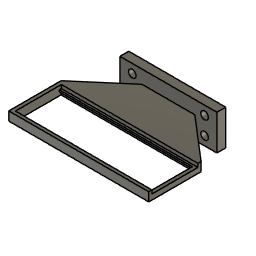
Specimen_slide_holder v2 (Autodesk Fusion 360 design; units mm, degrees)
Autodesk Fusion 360 part; units mm, degrees
note: some values were not read from the file. Set by a fixed rule: which sketch regions a step uses.
sketch "Sketch1" plane through (0, 0, 0) normal (0, 1, 0) x (1, 0, 0)
  line L0 (0, 0) -> (55, 0)
  line L1 (55, 0) -> (55, -20)
  line L2 (55, -20) -> (0, -20)
  line L3 (0, -20) -> (0, 0)
  line L4 (7, -20) -> (7, 0) construction
  line L5 (27.5, -20) -> (27.5, 0)
  line L6 (0, -10) -> (55, -10)
  line L7 (48, -20) -> (48, 0) construction
  line L8 (55, -15) -> (0, -15) construction
  circle A0 centre (7, -15) radius 2.15
  line L9 (55, -5) -> (0, -5) construction
  circle A1 centre (48, -15) radius 2.15
  circle A2 centre (7, -5) radius 2.15
  circle A3 centre (48, -5) radius 2.15
  line L10 (27.5, -10) -> (27.5, -12.5) construction
  line L11 (27.5, -12.5) -> (12.5, -12.5)
  line L12 (27.5, -12.5) -> (42.5, -12.5)
  line L13 (27.5, -7.5) -> (12.5, -7.5)
  line L14 (27.5, -7.5) -> (42.5, -7.5)
  line L15 (42.5, -12.5) -> (42.5, -7.5)
  line L16 (12.5, -12.5) -> (12.5, -7.5)
  dimension "d1" = 55
  dimension "d2" = 20
  dimension "d3" = 7
  dimension "d4" = 5
  dimension "d6" = 4.3
  dimension "d7" = 2.5
  dimension "d8" = 15
  dimension "d9" = 15
  constraint horizontal L0
  constraint vertical L1
  constraint horizontal L2
  constraint vertical L3
  constraint coincident L0.start L3.end
  constraint midpoint L2 L5.start
  constraint midpoint L0 L5.end
  constraint midpoint L3 L6.start
  constraint midpoint L1 L6.end
  constraint symmetric L4.start L5 L7.start
  constraint symmetric L4.end L5 L7.end
  constraint coincident L4 A0.centre
  constraint coincident L8 A0.centre
  constraint symmetric L6 L8.start L9.start
  constraint symmetric L6 L8.end L9.end
  constraint symmetric L5 A0 A1
  constraint symmetric L6 A0 A2
  constraint symmetric L6 A1 A3
  constraint midpoint L6 L10.start
  constraint perpendicular L2 L10
  constraint perpendicular L10 L11
  constraint perpendicular L10 L12
  constraint symmetric L6 L10.end L13.start
  constraint symmetric L6 L11.end L13.end
  constraint symmetric L6 L12.end L14.end
  measures "d1" distance of L0.start L0.end
  measures "d2" distance of L0.start L2.end
  measures "d6" diameter of A0
  measures "d7" distance of L10.start L10.end
  measures "d8" distance of L10.end L11.end
  measures "d9" distance of L10.end L12.end
extrude "Extrude1" add sketch "Sketch1" against normal blind 5 contours L0 L3 L5 L6 L13 L16 | L0 L1 L5 L6 L14 L15 | L2 L3 L5 L6 L11 L16 | L1 L2 L5 L6 L12 L15 makes body 1
extrude "Extrude2" add sketch "Sketch1" against normal blind 35 contours L5 L6 L14 L15 | L5 L6 L13 L16 | L5 L6 L11 L16 | L5 L6 L12 L15 bodies 1
ref_plane "WorkPlane1" through (27.5, -35, 10) normal (0, -1, 0) x (0, 0, -1)
sketch "Sketch2" plane through (0, -35, 0) normal (0, -1, 0) x (-1, 0, 0)
  line L0 (0, -20) -> (-55, -20) construction
  line L1 (-55, -20) -> (-55, 0) construction
  line L2 (-55, 0) -> (0, 0) construction
  line L3 (0, 0) -> (0, -20) construction
  line L4 (0, -10) -> (-55, -10)
  line L5 (-42.5, -12.5) -> (-42.5, -7.5) construction
  line L6 (-12.5, -7.5) -> (-12.5, -12.5) construction
  line L7 (-12.5, -12.5) -> (-42.5, -12.5) construction
  line L8 (-42.5, -7.5) -> (-12.5, -7.5) construction
  line L9 (-27.5, -20) -> (-27.5, 0) construction
  line L10 (-27.5, -10) -> (12.2, -10) construction
  line L11 (-27.5, -10) -> (-67.2, -10) construction
  line L12 (-27.5, -12.5) -> (12.2, -12.5)
  line L13 (-27.5, -12.5) -> (-67.2, -12.5)
  line L14 (-27.5, -7.5) -> (12.2, -7.5)
  line L15 (-27.5, -7.5) -> (-67.2, -7.5)
  line L16 (12.2, -12.5) -> (12.2, -7.5)
  line L17 (-67.2, -12.5) -> (-67.2, -7.5)
  line L18 (12.2, -12.5) -> (10.2, -12.5) construction
  line L19 (10.2, -12.5) -> (10.2, -7.5) construction
  line L20 (-67.2, -12.5) -> (-65.2, -12.5) construction
  line L21 (-65.2, -12.5) -> (-65.2, -7.5) construction
  point P0 (12.2, -12.5)
  dimension "d19" = 39.7
  dimension "d20" = 39.7
  dimension "d21" = 2.5
  dimension "d22" = 2
  dimension "d23" = 2
  constraint horizontal L0
  constraint vertical L1
  constraint horizontal L2
  constraint vertical L3
  constraint midpoint L3 L4.start
  constraint midpoint L1 L4.end
  constraint vertical L5
  constraint vertical L6
  constraint perpendicular L5 L7
  constraint perpendicular L6 L8
  constraint midpoint L0 L9.start
  constraint midpoint L2 L9.end
  constraint horizontal L10
  constraint midpoint L9 L10.start
  constraint perpendicular L9 L11
  constraint symmetric L4 L12.start L14.start
  constraint symmetric L4 P0 L14.end
  constraint symmetric L4 L13.end L15.end
  constraint perpendicular L16 L18
  constraint coincident L14 L19.end
  constraint perpendicular L14 L19
  constraint perpendicular L17 L20
  constraint coincident L15 L21.end
  constraint perpendicular L15 L21
  constraint coincident P0 L12.end
  measures "d19" distance of L10.start L10.end
  measures "d20" distance of L10.start L11.end
  measures "d22" distance of P0 L18.end
  measures "d23" distance of L13.end L20.end
ref_plane "WorkPlane2" through (27.5, -35, 7.5) normal (0, 0, 1) x (-1, 0, 0)
sketch "Sketch3" plane through (0, 0, 7.5) normal (0, 0, 1) x (1, 0, 0)
extrude "Extrude4" add sketch "Sketch2" along normal blind 29.7 bodies 1
sketch "Sketch4" plane through (0, 0, 12.5) normal (0, 0, 1) x (-1, 0, 0)
  line L0 (-42.5, 5) -> (-12.5, 5)
  line L1 (-12.5, 5) -> (-12.5, 35)
  line L2 (-12.5, 35) -> (12.2, 35)
  line L3 (12.2, 35) -> (12.2, 64.7)
  line L4 (12.2, 64.7) -> (-67.2, 64.7)
  line L5 (-67.2, 64.7) -> (-67.2, 35)
  line L6 (-67.2, 35) -> (-42.5, 35)
  line L7 (-42.5, 35) -> (-42.5, 5)
  line L8 (12.2, 35) -> (-67.2, 35) construction
  line L9 (-67.2, 35) -> (-67.2, 64.7) construction
  line L10 (-67.2, 64.7) -> (12.2, 64.7) construction
  line L11 (12.2, 64.7) -> (12.2, 35) construction
  line L12 (-65.2, 62.7) -> (10.2, 62.7)
  line L13 (10.2, 36) -> (-65.2, 36)
  line L14 (-27.5, 35) -> (-27.5, 64.7)
  line L15 (-65.2, 49.85) -> (10.2, 49.85)
  line L16 (10.25, 62.7) -> (10.25, 36)
  line L17 (10.25, 36) -> (10.2, 36)
  line L18 (10.25, 62.7) -> (10.2, 62.7)
  line L19 (-65.25, 62.7) -> (-65.25, 36)
  line L20 (-65.25, 62.7) -> (-65.2, 62.7)
  line L21 (-65.25, 36) -> (-65.2, 36)
  line L22 (-65.2, 61.7) -> (10.2, 61.7)
  line L23 (10.2, 61.7) -> (10.25, 61.7)
  line L24 (-65.2, 61.7) -> (-65.25, 61.7)
  line L25 (10.2, 37) -> (-65.2, 37)
  line L26 (10.2, 37) -> (10.25, 37)
  line L27 (-65.2, 37) -> (-65.25, 37)
  line L28 (10.2, 38) -> (10.25, 38)
  line L29 (-65.2, 38) -> (10.2, 38)
  line L30 (-65.2, 38) -> (-65.25, 38)
  line L31 (-65.25, 62.7) -> (-67.2, 62.7)
  line L32 (-65.25, 37) -> (-67.2, 37)
  line L33 (-42.5, 20) -> (-57.5, 35)
  line L34 (-27.5, 5) -> (-27.5, 34.5958)
  line L35 (-12.5, 20) -> (2.5, 35)
  dimension "d36" = 1
  dimension "d39" = 1
  constraint horizontal L8
  constraint vertical L9
  constraint horizontal L10
  constraint vertical L11
  constraint coincident L4.end L5.start
  constraint coincident L2.end L3.start
  constraint midpoint L8 L14.start
  constraint midpoint L10 L14.end
  constraint symmetric L13.start L14 L13.end
  constraint symmetric L12.end L14 L12.start
  constraint perpendicular L16 L17
  constraint perpendicular L16 L18
  constraint perpendicular L19 L20
  constraint perpendicular L19 L21
  constraint coincident L16 L23.end
  constraint perpendicular L16 L23
  constraint coincident L19 L24.end
  constraint perpendicular L19 L24
  constraint coincident L16 L26.end
  constraint perpendicular L16 L26
  constraint coincident L19 L27.end
  constraint perpendicular L19 L27
  constraint symmetric L15 L22.start L29.start
  constraint symmetric L15 L22.end L28.start
  constraint symmetric L15 L23.end L28.end
  constraint symmetric L15 L24.end L30.end
  constraint coincident L9 L31.end
  constraint perpendicular L9 L31
  constraint coincident L9 L32.end
  constraint perpendicular L9 L32
  constraint midpoint L7 L33.start
  constraint coincident L8 L33.end
  constraint midpoint L0 L34.start
  constraint perpendicular L8 L34
  constraint symmetric L33.start L34 L35.start
  constraint symmetric L33.end L34 L35.end
extrude "Extrude5" cut sketch "Sketch4" against normal blind 40 contours L13 L14 L19 L21 L25 L27 | L14 L19 L25 L27 L29 L30 | L12 L14 L19 L20 L22 L24 | L14 L19 L22 L24 L29 L30 | L13 L14 L16 L17 L25 L26 | L14 L16 L25 L26 L28 L29 | L12 L14 L16 L18 L22 L23 | L14 L16 L22 L23 L28 L29 bodies 1
extrude "Extrude6" add sketch "Sketch4" against normal blind 3.5 contours L13 L14 L19 L21 L25 L27 | L13 L14 L16 L17 L25 L26 bodies 1
extrude "Extrude7" add 1 faces at (40.0833, -36.6667, 9) along direction (0, 0, -1) blind 1.5 on bodies 1 bodies 1
extrude "Extrude8" add sketch "Sketch4" against normal blind 3.5 contours L14 L19 L25 L27 L29 L30 | L14 L16 L25 L26 L28 L29 bodies 1
extrude "Extrude9" cut sketch "Sketch4" against normal blind 2.5 contours L14 L19 L25 L27 L29 L30 | L14 L16 L25 L26 L28 L29 bodies 1
extrude "Extrude10" add sketch "Sketch4" against normal blind 3.5 contours L12 L14 L19 L20 L22 L24 | L12 L14 L16 L18 L22 L23 bodies 1
extrude "Extrude11" cut sketch "Sketch4" against normal blind 2.5 contours L12 L14 L19 L20 L22 L24 | L12 L14 L16 L18 L22 L23 bodies 1
sketch "Sketch5" plane through (67.2, 0, 0) normal (1, 0, 0) x (0, 1, 0)
  line L0 (-35, 7.5) -> (-35, 12.5)
  line L1 (-35, 12.5) -> (-64.7, 12.5)
  line L2 (-64.7, 12.5) -> (-64.7, 7.5)
  line L3 (-64.7, 7.5) -> (-35, 7.5)
  line L4 (-49.85, 12.5) -> (-49.85, 7.5)
  line L5 (-64.7, 10) -> (-35, 10)
  line L6 (-49.85, 10) -> (-49.85, 10.75) construction
  line L7 (-49.85, 10.75) -> (-62.7, 10.75)
  line L8 (-49.85, 9.25) -> (-62.7, 9.25)
  line L9 (-49.85, 10.75) -> (-37, 10.75)
  line L10 (-49.85, 9.25) -> (-37, 9.25)
  line L11 (-62.7, 10.75) -> (-62.7, 9.25)
  line L12 (-37, 10.75) -> (-37, 9.25)
  dimension "d51" = 0.75
  constraint midpoint L1 L4.start
  constraint midpoint L3 L4.end
  constraint midpoint L2 L5.start
  constraint midpoint L0 L5.end
  constraint midpoint L4 L6.start
  constraint perpendicular L5 L6
  constraint horizontal L7
  constraint symmetric L5 L6.end L8.start
  constraint symmetric L5 L7.end L8.end
  constraint symmetric L4 L6.end L7.start
  constraint symmetric L4 L7.end L9.end
  constraint symmetric L4 L8.start L10.start
  constraint symmetric L4 L8.end L10.end
  constraint perpendicular L8 L11
  measures "d51" distance of L6.start L6.end
extrude "Extrude12" cut sketch "Sketch5" against normal blind 2 contours L4 L5 L10 L12 | L4 L5 L9 L12 | L4 L5 L8 L11 | L4 L5 L7 L11 bodies 1
extrude "Extrude13" add 1 faces at (40.05, -62.3667, 10) along direction (0, 0, 1) blind 0.5 on bodies 1 bodies 1
extrude "Extrude14" cut 1 faces at (40.0833, -62.3667, 9) along direction (0, 0, 1) blind 0.5 on bodies 1 bodies 1
extrude "Extrude15" add 1 faces at (40.05, -37.3333, 10) along direction (0, 0, 1) blind 0.5 on bodies 1 bodies 1
extrude "Extrude16" cut 1 faces at (14.9167, -37.6667, 9) along direction (0, 0, 1) blind 0.5 on bodies 1 bodies 1
extrude "Extrude17" add 1 faces at (66.55, -45.5667, 9.25) along direction (0, 0, 1) blind 2 on bodies 1 bodies 1
extrude "Extrude18" cut sketch "Sketch4" against normal blind 2 contours L5 L19 L31 L32 bodies 1
extrude "Extrude19" add 1 faces at (65.2, -62.3667, 10.1667) along direction (1, 0, 0) blind 0.1 on bodies 1 bodies 1
extrude "Extrude20" add 1 faces at (65.2, -37.3333, 9.8333) along direction (1, 0, 0) blind 0.1 on bodies 1 bodies 1
extrude "Extrude21" cut 1 faces at (40.7167, -62.7, 11.8333) along direction (0, -1, 0) blind 0.1 on bodies 1 bodies 1
extrude "Extrude22" cut 1 faces at (40.0667, -37, 11.8333) along direction (0, 1, 0) blind 0.2 on bodies 1 bodies 1
extrude "Extrude23" cut 1 faces at (40.7167, -62.8, 11.8333) along direction (0, -1, 0) blind 0.1 on bodies 1 bodies 1
extrude "Extrude24" add sketch "Sketch4" against normal blind 5 contours L6 L7 L33 | L1 L2 L35 bodies 1
extrude "Extrude25" cut 1 faces at (42.5, -10, 10.8333) along direction (-1, 0, 0) blind 45 on bodies 1 bodies 1 makes body 2 at (33.6485, -5, 11.4554)
extrude "Extrude26" cut 1 faces at (32.5, -20, 10.8333) along direction (0, -1, 0) blind 15 on bodies 1 bodies 1
extrude "Extrude27" cut 1 faces at (42.5, -25, 10.8333) along direction (1, 0, 0) blind 35 on bodies 1 bodies 1
extrude "Extrude28" cut 1 faces at (12.5, -25, 10.8333) along direction (-1, 0, 0) blind 25 on bodies 1 bodies 1
move_body "Move1" bodies 1 to x (1, 0, 0) y (0, 1, 0) z (0, 0, 1) at (0, 8.835, 0)
extrude "Extrude29" add sketch "Sketch1" against normal blind 27 contours L5 L6 L14 L15 | L5 L6 L13 L16 | L5 L6 L11 L16 | L5 L6 L12 L15 bodies 1 2
sketch "Sketch6" plane through (0, 0, 12.5) normal (0, 0, 1) x (-1, 0, 0)
  line L0 (-12.5, 26.165) -> (12.2, 26.165)
  line L1 (12.2, 26.165) -> (12.2, 55.865)
  line L2 (12.2, 55.865) -> (-67.2, 55.865)
  line L3 (-67.2, 55.865) -> (-67.2, 54.065)
  line L4 (-67.2, 54.065) -> (10.25, 54.065)
  line L5 (10.25, 54.065) -> (10.25, 27.965)
  line L6 (10.25, 27.965) -> (-67.2, 27.965)
  line L7 (-67.2, 27.965) -> (-67.2, 26.165)
  line L8 (-67.2, 26.165) -> (-42.5, 26.165)
  line L9 (-42.5, 26.165) -> (-42.5, 5)
  line L10 (-42.5, 5) -> (-12.5, 5)
  line L11 (-12.5, 5) -> (-12.5, 26.165)
  line L12 (-67.2, 26.165) -> (-42.5, 5)
  line L13 (12.2, 26.165) -> (-12.5, 5)
  constraint coincident L7.end L8.start
  constraint coincident L9.end L10.start
  constraint coincident L0.end L1.start
  constraint coincident L10.end L11.start
extrude "Extrude30" add sketch "Sketch6" against normal blind 5 contours L0 L11 L13 | L8 L9 L12 bodies 1
extrude "Extrude3" [suppressed]
